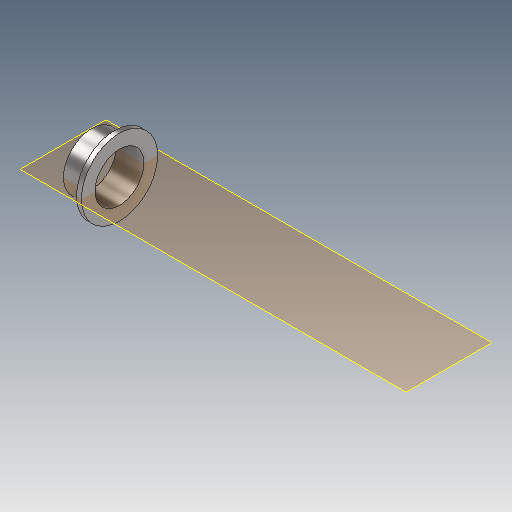
# Autodesk Inventor part: 低速轴套筒
Saved by Autodesk Inventor 2025 (Build 290162000, 162)
## iProperties
Created: 2025-03-20
Part Number: 低速轴套筒
Material: 钢，软
Document SubType Name: Modeling
Designer: liukan
Density: 7.85 g/cm^3
Appearance: 半抛光
Author: liukan
Autodesk Inventor part; units mm, degrees
ref_plane "YZ Plane" through (0, 0, 0) normal (1, 0, 0) x (0, 1, 0)
ref_plane "XZ Plane" through (0, 0, 0) normal (0, 1, 0) x (-1, 0, 0)
ref_plane "XY Plane" through (0, 0, 0) normal (0, 0, 1) x (1, 0, 0)
ref_plane "工作平面1" through (123.6693, 212.4733, -16.0979) normal (0, 1, 0) x (1, 0, 0)
sketch "草图1" plane through (123.6693, 212.4733, -16.0979) normal (0, 1, 0) x (1, 0, 0)
  line L0 (10.4501, 25) -> (10.4501, -25) projected
  line L1 (11.4501, 30.25) -> (11.4501, -30.25) projected
  line L2 (39.9501, 32) -> (39.9501, -32) projected
  line L3 (39.9501, -43) -> (39.9501, 43) projected
  line L4 (11.4501, -25) -> (39.9501, -25)
  line L5 (39.9501, -25) -> (39.9501, -29)
  line L6 (39.9501, -29) -> (11.4501, -29)
  line L7 (11.4501, -29) -> (11.4501, -25)
  line L8 (39.9501, -29) -> (34.9501, -29)
  line L9 (34.9501, -29) -> (34.9501, -39)
  line L10 (34.9501, -39) -> (39.9501, -39)
  line L11 (39.9501, -39) -> (39.9501, -29)
  line L12 (11.4501, 0) -> (39.9501, 0)
  point P0 (-123.6693, -16.0979)
  point P1 (34.9501, -29)
  dimension "d0" = 4
  dimension "d1" = 10
  dimension "d2" = 5
  constraints: 18 end point, 4 parallel, 3 point on line, 2 horizontal, 2 midpoint, 2 perpendicular
  measures "d0" distance of L4.end L5.end
  measures "d1" distance of L9.end L8.end
  measures "d2" distance of L9.end L10.end
revolve "旋转1" add sketch "草图1" angle 360 about axis through (135.1195, 212.4733, -16.0979) along (1, 0, 0) contours L4 L2 L6 L1 | L6 L2 L3 L10 L9
